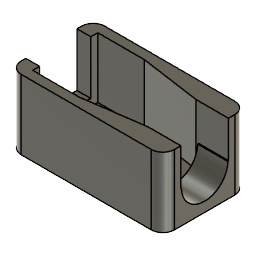
DC Barrel to Screw Terminal Adapter Fit Test (Autodesk Fusion 360 design; units mm, degrees)
Autodesk Fusion 360 part; units mm, degrees
sketch "Sketch1" plane through (0, 0, 0) normal (0, 0, 1) x (1, 0, 0)
  line L0 (0, 0) -> (0, 7)
  line L1 (0, 0) -> (0, -7)
  line L2 (0, 0) -> (20, 0)
  line L3 (20, 0) -> (20, -5.125)
  line L4 (20, 0) -> (20, 5.125)
  line L5 (0, 0) -> (13, 0)
  line L6 (20, 5.125) -> (13, 5.125)
  line L7 (13, 5.125) -> (13, -5.125)
  line L8 (13, -5.125) -> (20, -5.125)
  line L9 (20, -5.125) -> (20, 5.125)
  line L10 (0, 7) -> (13, 5.125)
  line L11 (0, -7) -> (13, -5.125)
  line L12 (0, 7) -> (-10, 7)
  line L13 (-10, 7) -> (-10, -7)
  line L14 (-10, -7) -> (0, -7)
  line L15 (0, -7) -> (0, 7)
  line L16 (-10, 0) -> (-10, 5.5)
  line L17 (-10, 0) -> (-10, -5.5)
  line L18 (20, -9) -> (0, -9)
  line L19 (0, -9) -> (0, 9)
  line L20 (0, 9) -> (20, 9)
  line L21 (20, 9) -> (20, -9)
  line L22 (20, -9) -> (0, 9) construction
  line L23 (0, -9) -> (20, 9) construction
  line L24 (-13, -9) -> (13, -9)
  line L25 (13, -9) -> (13, 9)
  line L26 (13, 9) -> (-13, 9)
  line L27 (-13, 9) -> (-13, -9)
  line L28 (-13, -9) -> (13, 9) construction
  line L29 (13, -9) -> (-13, 9) construction
  line L30 (-10, 5.5) -> (-13, 5.5)
  line L31 (-10, -5.5) -> (-13, -5.5)
  point P0 (10, 0)
  dimension "d1" = 7
  dimension "d2" = 5.125
  dimension "d3" = 5.125
  dimension "d4" = 13
  dimension "d5" = 5.5
  dimension "d6" = 5.5
  constraint coincident L0.start L1.start
  constraint vertical L0
  constraint parallel L0 L1
  constraint perpendicular L0 L2
  constraint perpendicular L2 L3
  constraint perpendicular L2 L4
  constraint perpendicular L0 L5
  constraint horizontal L6
  constraint vertical L7
  constraint horizontal L8
  constraint vertical L9
  constraint horizontal L12
  constraint vertical L13
  constraint horizontal L14
  constraint vertical L15
  constraint midpoint L13 L16.start
  constraint parallel L13 L16
  constraint parallel L13 L17
  constraint horizontal L18
  constraint perpendicular L18 L19
  constraint parallel L18 L20
  constraint parallel L19 L21
  constraint coincident L22 P0
  constraint coincident L23 P0
  constraint midpoint L2 P0
  constraint horizontal L24
  constraint perpendicular L24 L25
  constraint parallel L24 L26
  constraint parallel L25 L27
  constraint coincident L28 L0.start
  constraint coincident L29 L0.start
  constraint coincident L27 L30.end
  constraint perpendicular L27 L30
  constraint coincident L27 L31.end
  constraint perpendicular L27 L31
  measures "d1" distance of L0.start L0.end
  measures "d2" distance of L2.end L3.end
  measures "d3" distance of L2.end L4.end
  measures "d4" distance of L0.start L5.end
  measures "d5" distance of L16.start L16.end
  measures "d6" distance of L16.start L17.end
extrude "Extrude1" add sketch "Sketch1" along normal blind 15 contours L10 L19 L20 L25 L26 | L12 L13 L19 L26 L27 L30 | L13 L14 L19 L24 L27 L31 | L11 L18 L19 L24 L25 | L6 L20 L21 L25 | L8 L18 L21 L25 makes body 1 at (-2, -9, 5) makes body 2 at (-2, 9, 5)
extrude "Extrude2" add sketch "Sketch1" along normal blind 2 contours L0 L1 L12 L13 L14 L15 L16 L17 L19 | L1 L2 L5 L7 L11 L15 L19 L25 | L0 L2 L5 L7 L10 L15 L19 L25 | L2 L4 L6 L7 L9 L21 L25 | L2 L3 L7 L8 L9 L21 L25 bodies 1 2
extrude "Extrude3" add sketch "Sketch1" along normal blind 3.5 contours L13 L16 L17 L27 L30 L31 bodies 1
sketch "Sketch2" plane through (20, 0, 0) normal (1, 0, 0) x (0, 1, 0)
  line L0 (-9, 0) -> (9, 0)
  line L1 (9, 0) -> (9, 15)
  line L2 (9, 15) -> (5.125, 15)
  line L3 (5.125, 15) -> (5.125, 2)
  line L4 (5.125, 2) -> (-5.125, 2)
  line L5 (-5.125, 2) -> (-5.125, 15)
  line L6 (-5.125, 15) -> (-9, 15)
  line L7 (-9, 15) -> (-9, 0)
  line L8 (0, 2) -> (0, 7.1)
  circle A0 centre (0, 7.1) radius 5
  line L9 (-5, 7.1) -> (-5.125, 7.1)
  line L10 (5, 7.1) -> (5.125, 7.1)
  dimension "d13" = 5.1
  dimension "d14" = 10
  constraint midpoint L4 L8.start
  constraint perpendicular L4 L8
  constraint coincident L8.end A0.centre
  constraint coincident A0 L9.start
  constraint coincident L5 L9.end
  constraint perpendicular L5 L9
  constraint coincident A0 L10.start
  constraint coincident L3 L10.end
  constraint perpendicular L3 L10
  measures "d13" distance of L8.start L8.end
  measures "d14" diameter of A0
extrude "Extrude4" add sketch "Sketch2" against normal blind 6.5 contours L4 L5 L8 A0 L9 | L3 L4 L8 A0 L10 bodies 1
chamfer "Chamfer1" distance 0.1 angle 45 2 edges at (16.75, -5, 7.1) (16.75, 5, 7.1) on bodies 1
fillet "Fillet1" radius 2.5 4 edges at (-13, -9, 7.5) (20, -9, 7.5) (-13, 9, 7.5) (20, 9, 7.5) on bodies 1
